Autodesk Inventor part; units mm, degrees
(part 4 of 6)
  line L2768 (19.2612, 25.2556) -> (20.2612, 25.2556)
  line L2769 (20.2612, 25.2556) -> (20.2612, 26.2556)
  line L2770 (20.2612, 26.2556) -> (19.2612, 26.2556)
  line L2771 (19.2612, 26.2556) -> (19.2612, 25.2556)
  line L2772 (19.8708, 25.2556) -> (20.8708, 25.2556)
  line L2773 (20.8708, 25.2556) -> (20.8708, 26.2556)
  line L2774 (20.8708, 26.2556) -> (19.8708, 26.2556)
  line L2775 (19.8708, 26.2556) -> (19.8708, 25.2556)
  line L2776 (20.4804, 25.2556) -> (21.4804, 25.2556)
  line L2777 (21.4804, 25.2556) -> (21.4804, 26.2556)
  line L2778 (21.4804, 26.2556) -> (20.4804, 26.2556)
  line L2779 (20.4804, 26.2556) -> (20.4804, 25.2556)
  line L2780 (21.2678, 25.2556) -> (22.2678, 25.2556)
  line L2781 (22.2678, 25.2556) -> (22.2678, 26.2556)
  line L2782 (22.2678, 26.2556) -> (21.2678, 26.2556)
  line L2783 (21.2678, 26.2556) -> (21.2678, 25.2556)
  line L2784 (21.7504, 25.2556) -> (22.7504, 25.2556)
  line L2785 (22.7504, 25.2556) -> (22.7504, 26.2556)
  line L2786 (22.7504, 26.2556) -> (21.7504, 26.2556)
  line L2787 (21.7504, 26.2556) -> (21.7504, 25.2556)
  line L2788 (12.8731, 25.281) -> (13.8731, 25.281)
  line L2789 (13.8731, 25.281) -> (13.8731, 26.281)
  line L2790 (13.8731, 26.281) -> (12.8731, 26.281)
  line L2791 (12.8731, 26.281) -> (12.8731, 25.281)
  line L2792 (14.5749, 25.281) -> (15.5749, 25.281)
  line L2793 (15.5749, 25.281) -> (15.5749, 26.281)
  line L2794 (15.5749, 26.281) -> (14.5749, 26.281)
  line L2795 (14.5749, 26.281) -> (14.5749, 25.281)
  line L2796 (15.4893, 25.281) -> (16.4893, 25.281)
  line L2797 (16.4893, 25.281) -> (16.4893, 26.281)
  line L2798 (16.4893, 26.281) -> (15.4893, 26.281)
  line L2799 (15.4893, 26.281) -> (15.4893, 25.281)
  line L2800 (16.2386, 25.281) -> (17.2386, 25.281)
  line L2801 (17.2386, 25.281) -> (17.2386, 26.281)
  line L2802 (17.2386, 26.281) -> (16.2386, 26.281)
  line L2803 (16.2386, 26.281) -> (16.2386, 25.281)
  line L2804 (17.0768, 25.281) -> (18.0768, 25.281)
  line L2805 (18.0768, 25.281) -> (18.0768, 26.281)
  line L2806 (18.0768, 26.281) -> (17.0768, 26.281)
  line L2807 (17.0768, 26.281) -> (17.0768, 25.281)
  line L2808 (17.9658, 25.281) -> (18.9658, 25.281)
  line L2809 (18.9658, 25.281) -> (18.9658, 26.281)
  line L2810 (18.9658, 26.281) -> (17.9658, 26.281)
  line L2811 (17.9658, 26.281) -> (17.9658, 25.281)
  line L2812 (18.6897, 25.281) -> (19.6897, 25.281)
  line L2813 (19.6897, 25.281) -> (19.6897, 26.281)
  line L2814 (19.6897, 26.281) -> (18.6897, 26.281)
  line L2815 (18.6897, 26.281) -> (18.6897, 25.281)
  line L2816 (19.2739, 25.281) -> (20.2739, 25.281)
  line L2817 (20.2739, 25.281) -> (20.2739, 26.281)
  line L2818 (20.2739, 26.281) -> (19.2739, 26.281)
  line L2819 (19.2739, 26.281) -> (19.2739, 25.281)
  line L2820 (19.8708, 25.281) -> (20.8708, 25.281)
  line L2821 (20.8708, 25.281) -> (20.8708, 26.281)
  line L2822 (20.8708, 26.281) -> (19.8708, 26.281)
  line L2823 (19.8708, 26.281) -> (19.8708, 25.281)
  line L2824 (20.4804, 25.281) -> (21.4804, 25.281)
  line L2825 (21.4804, 25.281) -> (21.4804, 26.281)
  line L2826 (21.4804, 26.281) -> (20.4804, 26.281)
  line L2827 (20.4804, 26.281) -> (20.4804, 25.281)
  line L2828 (21.2424, 25.281) -> (22.2424, 25.281)
  line L2829 (22.2424, 25.281) -> (22.2424, 26.281)
  line L2830 (22.2424, 26.281) -> (21.2424, 26.281)
  line L2831 (21.2424, 26.281) -> (21.2424, 25.281)
  line L2832 (21.7758, 25.281) -> (22.7758, 25.281)
  line L2833 (22.7758, 25.281) -> (22.7758, 26.281)
  line L2834 (22.7758, 26.281) -> (21.7758, 26.281)
  line L2835 (21.7758, 26.281) -> (21.7758, 25.281)
  line L2836 (12.8985, 25.3064) -> (13.8985, 25.3064)
  line L2837 (13.8985, 25.3064) -> (13.8985, 26.3064)
  line L2838 (13.8985, 26.3064) -> (12.8985, 26.3064)
  line L2839 (12.8985, 26.3064) -> (12.8985, 25.3064)
  line L2840 (14.6003, 25.3064) -> (15.6003, 25.3064)
  line L2841 (15.6003, 25.3064) -> (15.6003, 26.3064)
  line L2842 (15.6003, 26.3064) -> (14.6003, 26.3064)
  line L2843 (14.6003, 26.3064) -> (14.6003, 25.3064)
  line L2844 (15.502, 25.3064) -> (16.502, 25.3064)
  line L2845 (16.502, 25.3064) -> (16.502, 26.3064)
  line L2846 (16.502, 26.3064) -> (15.502, 26.3064)
  line L2847 (15.502, 26.3064) -> (15.502, 25.3064)
  line L2848 (16.2386, 25.3064) -> (17.2386, 25.3064)
  line L2849 (17.2386, 25.3064) -> (17.2386, 26.3064)
  line L2850 (17.2386, 26.3064) -> (16.2386, 26.3064)
  line L2851 (16.2386, 26.3064) -> (16.2386, 25.3064)
  line L2852 (17.0768, 25.3064) -> (18.0768, 25.3064)
  line L2853 (18.0768, 25.3064) -> (18.0768, 26.3064)
  line L2854 (18.0768, 26.3064) -> (17.0768, 26.3064)
  line L2855 (17.0768, 26.3064) -> (17.0768, 25.3064)
  line L2856 (17.9658, 25.3064) -> (18.9658, 25.3064)
  line L2857 (18.9658, 25.3064) -> (18.9658, 26.3064)
  line L2858 (18.9658, 26.3064) -> (17.9658, 26.3064)
  line L2859 (17.9658, 26.3064) -> (17.9658, 25.3064)
  line L2860 (18.677, 25.3064) -> (19.677, 25.3064)
  line L2861 (19.677, 25.3064) -> (19.677, 26.3064)
  line L2862 (19.677, 26.3064) -> (18.677, 26.3064)
  line L2863 (18.677, 26.3064) -> (18.677, 25.3064)
  line L2864 (19.2739, 25.3064) -> (20.2739, 25.3064)
  line L2865 (20.2739, 25.3064) -> (20.2739, 26.3064)
  line L2866 (20.2739, 26.3064) -> (19.2739, 26.3064)
  line L2867 (19.2739, 26.3064) -> (19.2739, 25.3064)
  line L2868 (19.7057, 25.3064) -> (20.7057, 25.3064)
  line L2869 (20.7057, 25.3064) -> (20.7057, 26.3064)
  line L2870 (20.7057, 26.3064) -> (19.7057, 26.3064)
  line L2871 (19.7057, 26.3064) -> (19.7057, 25.3064)
  line L2872 (20.0486, 25.3064) -> (21.0486, 25.3064)
  line L2873 (21.0486, 25.3064) -> (21.0486, 26.3064)
  line L2874 (21.0486, 26.3064) -> (20.0486, 26.3064)
  line L2875 (20.0486, 26.3064) -> (20.0486, 25.3064)
  line L2876 (20.4804, 25.3064) -> (21.4804, 25.3064)
  line L2877 (21.4804, 25.3064) -> (21.4804, 26.3064)
  line L2878 (21.4804, 26.3064) -> (20.4804, 26.3064)
  line L2879 (20.4804, 26.3064) -> (20.4804, 25.3064)
  line L2880 (21.2424, 25.3064) -> (22.2424, 25.3064)
  line L2881 (22.2424, 25.3064) -> (22.2424, 26.3064)
  line L2882 (22.2424, 26.3064) -> (21.2424, 26.3064)
  line L2883 (21.2424, 26.3064) -> (21.2424, 25.3064)
  line L2884 (21.7758, 25.3064) -> (22.7758, 25.3064)
  line L2885 (22.7758, 25.3064) -> (22.7758, 26.3064)
  line L2886 (22.7758, 26.3064) -> (21.7758, 26.3064)
  line L2887 (21.7758, 26.3064) -> (21.7758, 25.3064)
  line L2888 (12.9239, 25.3318) -> (13.9239, 25.3318)
  line L2889 (13.9239, 25.3318) -> (13.9239, 26.3318)
  line L2890 (13.9239, 26.3318) -> (12.9239, 26.3318)
  line L2891 (12.9239, 26.3318) -> (12.9239, 25.3318)
  line L2892 (14.6257, 25.3318) -> (15.6257, 25.3318)
  line L2893 (15.6257, 25.3318) -> (15.6257, 26.3318)
  line L2894 (15.6257, 26.3318) -> (14.6257, 26.3318)
  line L2895 (14.6257, 26.3318) -> (14.6257, 25.3318)
  line L2896 (15.502, 25.3318) -> (16.502, 25.3318)
  line L2897 (16.502, 25.3318) -> (16.502, 26.3318)
  line L2898 (16.502, 26.3318) -> (15.502, 26.3318)
  line L2899 (15.502, 26.3318) -> (15.502, 25.3318)
  line L2900 (16.2386, 25.3318) -> (17.2386, 25.3318)
  line L2901 (17.2386, 25.3318) -> (17.2386, 26.3318)
  line L2902 (17.2386, 26.3318) -> (16.2386, 26.3318)
  line L2903 (16.2386, 26.3318) -> (16.2386, 25.3318)
  line L2904 (17.0768, 25.3318) -> (18.0768, 25.3318)
  line L2905 (18.0768, 25.3318) -> (18.0768, 26.3318)
  line L2906 (18.0768, 26.3318) -> (17.0768, 26.3318)
  line L2907 (17.0768, 26.3318) -> (17.0768, 25.3318)
  line L2908 (17.9785, 25.3318) -> (18.9785, 25.3318)
  line L2909 (18.9785, 25.3318) -> (18.9785, 26.3318)
  line L2910 (18.9785, 26.3318) -> (17.9785, 26.3318)
  line L2911 (17.9785, 26.3318) -> (17.9785, 25.3318)
  line L2912 (18.6897, 25.3318) -> (19.6897, 25.3318)
  line L2913 (19.6897, 25.3318) -> (19.6897, 26.3318)
  line L2914 (19.6897, 26.3318) -> (18.6897, 26.3318)
  line L2915 (18.6897, 26.3318) -> (18.6897, 25.3318)
  line L2916 (19.2739, 25.3318) -> (20.2739, 25.3318)
  line L2917 (20.2739, 25.3318) -> (20.2739, 26.3318)
  line L2918 (20.2739, 26.3318) -> (19.2739, 26.3318)
  line L2919 (19.2739, 26.3318) -> (19.2739, 25.3318)
  line L2920 (19.693, 25.3318) -> (20.693, 25.3318)
  line L2921 (20.693, 25.3318) -> (20.693, 26.3318)
  line L2922 (20.693, 26.3318) -> (19.693, 26.3318)
  line L2923 (19.693, 26.3318) -> (19.693, 25.3318)
  line L2924 (20.0613, 25.3318) -> (21.0613, 25.3318)
  line L2925 (21.0613, 25.3318) -> (21.0613, 26.3318)
  line L2926 (21.0613, 26.3318) -> (20.0613, 26.3318)
  line L2927 (20.0613, 26.3318) -> (20.0613, 25.3318)
  line L2928 (20.4804, 25.3318) -> (21.4804, 25.3318)
  line L2929 (21.4804, 25.3318) -> (21.4804, 26.3318)
  line L2930 (21.4804, 26.3318) -> (20.4804, 26.3318)
  line L2931 (20.4804, 26.3318) -> (20.4804, 25.3318)
  line L2932 (21.2297, 25.3318) -> (22.2297, 25.3318)
  line L2933 (22.2297, 25.3318) -> (22.2297, 26.3318)
  line L2934 (22.2297, 26.3318) -> (21.2297, 26.3318)
  line L2935 (21.2297, 26.3318) -> (21.2297, 25.3318)
  line L2936 (21.8012, 25.3318) -> (22.8012, 25.3318)
  line L2937 (22.8012, 25.3318) -> (22.8012, 26.3318)
  line L2938 (22.8012, 26.3318) -> (21.8012, 26.3318)
  line L2939 (21.8012, 26.3318) -> (21.8012, 25.3318)
  line L2940 (12.9366, 25.3572) -> (13.9366, 25.3572)
  line L2941 (13.9366, 25.3572) -> (13.9366, 26.3572)
  line L2942 (13.9366, 26.3572) -> (12.9366, 26.3572)
  line L2943 (12.9366, 26.3572) -> (12.9366, 25.3572)
  line L2944 (14.6511, 25.3572) -> (15.6511, 25.3572)
  line L2945 (15.6511, 25.3572) -> (15.6511, 26.3572)
  line L2946 (15.6511, 26.3572) -> (14.6511, 26.3572)
  line L2947 (14.6511, 26.3572) -> (14.6511, 25.3572)
  line L2948 (15.502, 25.3572) -> (16.502, 25.3572)
  line L2949 (16.502, 25.3572) -> (16.502, 26.3572)
  line L2950 (16.502, 26.3572) -> (15.502, 26.3572)
  line L2951 (15.502, 26.3572) -> (15.502, 25.3572)
  line L2952 (16.2386, 25.3572) -> (17.2386, 25.3572)
  line L2953 (17.2386, 25.3572) -> (17.2386, 26.3572)
  line L2954 (17.2386, 26.3572) -> (16.2386, 26.3572)
  line L2955 (16.2386, 26.3572) -> (16.2386, 25.3572)
  line L2956 (16.7466, 25.3572) -> (17.7466, 25.3572)
  line L2957 (17.7466, 25.3572) -> (17.7466, 26.3572)
  line L2958 (17.7466, 26.3572) -> (16.7466, 26.3572)
  line L2959 (16.7466, 26.3572) -> (16.7466, 25.3572)
  line L2960 (17.4197, 25.3572) -> (18.4197, 25.3572)
  line L2961 (18.4197, 25.3572) -> (18.4197, 26.3572)
  line L2962 (18.4197, 26.3572) -> (17.4197, 26.3572)
  line L2963 (17.4197, 26.3572) -> (17.4197, 25.3572)
  line L2964 (17.9785, 25.3572) -> (18.9785, 25.3572)
  line L2965 (18.9785, 25.3572) -> (18.9785, 26.3572)
  line L2966 (18.9785, 26.3572) -> (17.9785, 26.3572)
  line L2967 (17.9785, 26.3572) -> (17.9785, 25.3572)
  line L2968 (18.6897, 25.3572) -> (19.6897, 25.3572)
  line L2969 (19.6897, 25.3572) -> (19.6897, 26.3572)
  line L2970 (19.6897, 26.3572) -> (18.6897, 26.3572)
  line L2971 (18.6897, 26.3572) -> (18.6897, 25.3572)
  line L2972 (19.2739, 25.3572) -> (20.2739, 25.3572)
  line L2973 (20.2739, 25.3572) -> (20.2739, 26.3572)
  line L2974 (20.2739, 26.3572) -> (19.2739, 26.3572)
  line L2975 (19.2739, 26.3572) -> (19.2739, 25.3572)
  line L2976 (19.693, 25.3572) -> (20.693, 25.3572)
  line L2977 (20.693, 25.3572) -> (20.693, 26.3572)
  line L2978 (20.693, 26.3572) -> (19.693, 26.3572)
  line L2979 (19.693, 26.3572) -> (19.693, 25.3572)
  line L2980 (20.0613, 25.3572) -> (21.0613, 25.3572)
  line L2981 (21.0613, 25.3572) -> (21.0613, 26.3572)
  line L2982 (21.0613, 26.3572) -> (20.0613, 26.3572)
  line L2983 (20.0613, 26.3572) -> (20.0613, 25.3572)
  line L2984 (20.4931, 25.3572) -> (21.4931, 25.3572)
  line L2985 (21.4931, 25.3572) -> (21.4931, 26.3572)
  line L2986 (21.4931, 26.3572) -> (20.4931, 26.3572)
  line L2987 (20.4931, 26.3572) -> (20.4931, 25.3572)
  line L2988 (21.217, 25.3572) -> (22.217, 25.3572)
  line L2989 (22.217, 25.3572) -> (22.217, 26.3572)
  line L2990 (22.217, 26.3572) -> (21.217, 26.3572)
  line L2991 (21.217, 26.3572) -> (21.217, 25.3572)
  line L2992 (21.8012, 25.3572) -> (22.8012, 25.3572)
  line L2993 (22.8012, 25.3572) -> (22.8012, 26.3572)
  line L2994 (22.8012, 26.3572) -> (21.8012, 26.3572)
  line L2995 (21.8012, 26.3572) -> (21.8012, 25.3572)
  line L2996 (12.962, 25.3826) -> (13.962, 25.3826)
  line L2997 (13.962, 25.3826) -> (13.962, 26.3826)
  line L2998 (13.962, 26.3826) -> (12.962, 26.3826)
  line L2999 (12.962, 26.3826) -> (12.962, 25.3826)
  line L3000 (14.6765, 25.3826) -> (15.6765, 25.3826)
  line L3001 (15.6765, 25.3826) -> (15.6765, 26.3826)
  line L3002 (15.6765, 26.3826) -> (14.6765, 26.3826)
  line L3003 (14.6765, 26.3826) -> (14.6765, 25.3826)
  line L3004 (15.5147, 25.3826) -> (16.5147, 25.3826)
  line L3005 (16.5147, 25.3826) -> (16.5147, 26.3826)
  line L3006 (16.5147, 26.3826) -> (15.5147, 26.3826)
  line L3007 (15.5147, 26.3826) -> (15.5147, 25.3826)
  line L3008 (16.2259, 25.3826) -> (17.2259, 25.3826)
  line L3009 (17.2259, 25.3826) -> (17.2259, 26.3826)
  line L3010 (17.2259, 26.3826) -> (16.2259, 26.3826)
  line L3011 (16.2259, 26.3826) -> (16.2259, 25.3826)
  line L3012 (16.7593, 25.3826) -> (17.7593, 25.3826)
  line L3013 (17.7593, 25.3826) -> (17.7593, 26.3826)
  line L3014 (17.7593, 26.3826) -> (16.7593, 26.3826)
  line L3015 (16.7593, 26.3826) -> (16.7593, 25.3826)
  line L3016 (17.4197, 25.3826) -> (18.4197, 25.3826)
  line L3017 (18.4197, 25.3826) -> (18.4197, 26.3826)
  line L3018 (18.4197, 26.3826) -> (17.4197, 26.3826)
  line L3019 (17.4197, 26.3826) -> (17.4197, 25.3826)
  line L3020 (17.9912, 25.3826) -> (18.9912, 25.3826)
  line L3021 (18.9912, 25.3826) -> (18.9912, 26.3826)
  line L3022 (18.9912, 26.3826) -> (17.9912, 26.3826)
  line L3023 (17.9912, 26.3826) -> (17.9912, 25.3826)
  line L3024 (18.6897, 25.3826) -> (19.6897, 25.3826)
  line L3025 (19.6897, 25.3826) -> (19.6897, 26.3826)
  line L3026 (19.6897, 26.3826) -> (18.6897, 26.3826)
  line L3027 (18.6897, 26.3826) -> (18.6897, 25.3826)
  line L3028 (19.2739, 25.3826) -> (20.2739, 25.3826)
  line L3029 (20.2739, 25.3826) -> (20.2739, 26.3826)
  line L3030 (20.2739, 26.3826) -> (19.2739, 26.3826)
  line L3031 (19.2739, 26.3826) -> (19.2739, 25.3826)
  line L3032 (19.693, 25.3826) -> (20.693, 25.3826)
  line L3033 (20.693, 25.3826) -> (20.693, 26.3826)
  line L3034 (20.693, 26.3826) -> (19.693, 26.3826)
  line L3035 (19.693, 26.3826) -> (19.693, 25.3826)
  line L3036 (20.0613, 25.3826) -> (21.0613, 25.3826)
  line L3037 (21.0613, 25.3826) -> (21.0613, 26.3826)
  line L3038 (21.0613, 26.3826) -> (20.0613, 26.3826)
  line L3039 (20.0613, 26.3826) -> (20.0613, 25.3826)
  line L3040 (20.4931, 25.3826) -> (21.4931, 25.3826)
  line L3041 (21.4931, 25.3826) -> (21.4931, 26.3826)
  line L3042 (21.4931, 26.3826) -> (20.4931, 26.3826)
  line L3043 (20.4931, 26.3826) -> (20.4931, 25.3826)
  line L3044 (21.217, 25.3826) -> (22.217, 25.3826)
  line L3045 (22.217, 25.3826) -> (22.217, 26.3826)
  line L3046 (22.217, 26.3826) -> (21.217, 26.3826)
  line L3047 (21.217, 26.3826) -> (21.217, 25.3826)
  line L3048 (21.8266, 25.3826) -> (22.8266, 25.3826)
  line L3049 (22.8266, 25.3826) -> (22.8266, 26.3826)
  line L3050 (22.8266, 26.3826) -> (21.8266, 26.3826)
  line L3051 (21.8266, 26.3826) -> (21.8266, 25.3826)
  line L3052 (12.9874, 25.408) -> (13.9874, 25.408)
  line L3053 (13.9874, 25.408) -> (13.9874, 26.408)
  line L3054 (13.9874, 26.408) -> (12.9874, 26.408)
  line L3055 (12.9874, 26.408) -> (12.9874, 25.408)
  line L3056 (14.7019, 25.408) -> (15.7019, 25.408)
  line L3057 (15.7019, 25.408) -> (15.7019, 26.408)
  line L3058 (15.7019, 26.408) -> (14.7019, 26.408)
  line L3059 (14.7019, 26.408) -> (14.7019, 25.408)
  line L3060 (15.5147, 25.408) -> (16.5147, 25.408)
  line L3061 (16.5147, 25.408) -> (16.5147, 26.408)
  line L3062 (16.5147, 26.408) -> (15.5147, 26.408)
  line L3063 (15.5147, 26.408) -> (15.5147, 25.408)
  line L3064 (16.2132, 25.408) -> (17.2132, 25.408)
  line L3065 (17.2132, 25.408) -> (17.2132, 26.408)
  line L3066 (17.2132, 26.408) -> (16.2132, 26.408)
  line L3067 (16.2132, 26.408) -> (16.2132, 25.408)
  line L3068 (16.7593, 25.408) -> (17.7593, 25.408)
  line L3069 (17.7593, 25.408) -> (17.7593, 26.408)
  line L3070 (17.7593, 26.408) -> (16.7593, 26.408)
  line L3071 (16.7593, 26.408) -> (16.7593, 25.408)
  line L3072 (17.4197, 25.408) -> (18.4197, 25.408)
  line L3073 (18.4197, 25.408) -> (18.4197, 26.408)
  line L3074 (18.4197, 26.408) -> (17.4197, 26.408)
  line L3075 (17.4197, 26.408) -> (17.4197, 25.408)
  line L3076 (18.0039, 25.408) -> (19.0039, 25.408)
  line L3077 (19.0039, 25.408) -> (19.0039, 26.408)
  line L3078 (19.0039, 26.408) -> (18.0039, 26.408)
  line L3079 (18.0039, 26.408) -> (18.0039, 25.408)
  line L3080 (18.677, 25.408) -> (19.677, 25.408)
  line L3081 (19.677, 25.408) -> (19.677, 26.408)
  line L3082 (19.677, 26.408) -> (18.677, 26.408)
  line L3083 (18.677, 26.408) -> (18.677, 25.408)
  line L3084 (19.2739, 25.408) -> (20.2739, 25.408)
  line L3085 (20.2739, 25.408) -> (20.2739, 26.408)
  line L3086 (20.2739, 26.408) -> (19.2739, 26.408)
  line L3087 (19.2739, 26.408) -> (19.2739, 25.408)
  line L3088 (19.693, 25.408) -> (20.693, 25.408)
  line L3089 (20.693, 25.408) -> (20.693, 26.408)
  line L3090 (20.693, 26.408) -> (19.693, 26.408)
  line L3091 (19.693, 26.408) -> (19.693, 25.408)
  line L3092 (20.0867, 25.408) -> (21.0867, 25.408)
  line L3093 (21.0867, 25.408) -> (21.0867, 26.408)
  line L3094 (21.0867, 26.408) -> (20.0867, 26.408)
  line L3095 (20.0867, 26.408) -> (20.0867, 25.408)
  line L3096 (20.4931, 25.408) -> (21.4931, 25.408)
  line L3097 (21.4931, 25.408) -> (21.4931, 26.408)
  line L3098 (21.4931, 26.408) -> (20.4931, 26.408)
  line L3099 (20.4931, 26.408) -> (20.4931, 25.408)
  line L3100 (21.2043, 25.408) -> (22.2043, 25.408)
  line L3101 (22.2043, 25.408) -> (22.2043, 26.408)
  line L3102 (22.2043, 26.408) -> (21.2043, 26.408)
  line L3103 (21.2043, 26.408) -> (21.2043, 25.408)
  line L3104 (21.8266, 25.408) -> (22.8266, 25.408)
  line L3105 (22.8266, 25.408) -> (22.8266, 26.408)
  line L3106 (22.8266, 26.408) -> (21.8266, 26.408)
  line L3107 (21.8266, 26.408) -> (21.8266, 25.408)
  line L3108 (13.0128, 25.4334) -> (14.0128, 25.4334)
  line L3109 (14.0128, 25.4334) -> (14.0128, 26.4334)
  line L3110 (14.0128, 26.4334) -> (13.0128, 26.4334)
  line L3111 (13.0128, 26.4334) -> (13.0128, 25.4334)
  line L3112 (14.7273, 25.4334) -> (15.7273, 25.4334)
  line L3113 (15.7273, 25.4334) -> (15.7273, 26.4334)
  line L3114 (15.7273, 26.4334) -> (14.7273, 26.4334)
  line L3115 (14.7273, 26.4334) -> (14.7273, 25.4334)
  line L3116 (15.5147, 25.4334) -> (16.5147, 25.4334)
  line L3117 (16.5147, 25.4334) -> (16.5147, 26.4334)
  line L3118 (16.5147, 26.4334) -> (15.5147, 26.4334)
  line L3119 (15.5147, 26.4334) -> (15.5147, 25.4334)
  line L3120 (16.2005, 25.4334) -> (17.2005, 25.4334)
  line L3121 (17.2005, 25.4334) -> (17.2005, 26.4334)
  line L3122 (17.2005, 26.4334) -> (16.2005, 26.4334)
  line L3123 (16.2005, 26.4334) -> (16.2005, 25.4334)
  line L3124 (16.7593, 25.4334) -> (17.7593, 25.4334)
  line L3125 (17.7593, 25.4334) -> (17.7593, 26.4334)
  line L3126 (17.7593, 26.4334) -> (16.7593, 26.4334)
  line L3127 (16.7593, 26.4334) -> (16.7593, 25.4334)
  line L3128 (17.4197, 25.4334) -> (18.4197, 25.4334)
  line L3129 (18.4197, 25.4334) -> (18.4197, 26.4334)
  line L3130 (18.4197, 26.4334) -> (17.4197, 26.4334)
  line L3131 (17.4197, 26.4334) -> (17.4197, 25.4334)
  line L3132 (18.0166, 25.4334) -> (19.0166, 25.4334)
  line L3133 (19.0166, 25.4334) -> (19.0166, 26.4334)
  line L3134 (19.0166, 26.4334) -> (18.0166, 26.4334)
  line L3135 (18.0166, 26.4334) -> (18.0166, 25.4334)
  line L3136 (18.6643, 25.4334) -> (19.6643, 25.4334)
  line L3137 (19.6643, 25.4334) -> (19.6643, 26.4334)
  line L3138 (19.6643, 26.4334) -> (18.6643, 26.4334)
  line L3139 (18.6643, 26.4334) -> (18.6643, 25.4334)
  line L3140 (19.2739, 25.4334) -> (20.2739, 25.4334)
  line L3141 (20.2739, 25.4334) -> (20.2739, 26.4334)
  line L3142 (20.2739, 26.4334) -> (19.2739, 26.4334)
  line L3143 (19.2739, 26.4334) -> (19.2739, 25.4334)
  line L3144 (19.6676, 25.4334) -> (20.6676, 25.4334)
  line L3145 (20.6676, 25.4334) -> (20.6676, 26.4334)
  line L3146 (20.6676, 26.4334) -> (19.6676, 26.4334)
  line L3147 (19.6676, 26.4334) -> (19.6676, 25.4334)
  line L3148 (20.0867, 25.4334) -> (21.0867, 25.4334)
  line L3149 (21.0867, 25.4334) -> (21.0867, 26.4334)
  line L3150 (21.0867, 26.4334) -> (20.0867, 26.4334)
  line L3151 (20.0867, 26.4334) -> (20.0867, 25.4334)
  line L3152 (20.4931, 25.4334) -> (21.4931, 25.4334)
  line L3153 (21.4931, 25.4334) -> (21.4931, 26.4334)
  line L3154 (21.4931, 26.4334) -> (20.4931, 26.4334)
  line L3155 (20.4931, 26.4334) -> (20.4931, 25.4334)
  line L3156 (21.1916, 25.4334) -> (22.1916, 25.4334)
  line L3157 (22.1916, 25.4334) -> (22.1916, 26.4334)
  line L3158 (22.1916, 26.4334) -> (21.1916, 26.4334)
  line L3159 (21.1916, 26.4334) -> (21.1916, 25.4334)
  line L3160 (21.8393, 25.4334) -> (22.8393, 25.4334)
  line L3161 (22.8393, 25.4334) -> (22.8393, 26.4334)
  line L3162 (22.8393, 26.4334) -> (21.8393, 26.4334)
  line L3163 (21.8393, 26.4334) -> (21.8393, 25.4334)
  line L3164 (13.0255, 25.4588) -> (14.0255, 25.4588)
  line L3165 (14.0255, 25.4588) -> (14.0255, 26.4588)
  line L3166 (14.0255, 26.4588) -> (13.0255, 26.4588)
  line L3167 (13.0255, 26.4588) -> (13.0255, 25.4588)
  line L3168 (14.74, 25.4588) -> (15.74, 25.4588)
  line L3169 (15.74, 25.4588) -> (15.74, 26.4588)
  line L3170 (15.74, 26.4588) -> (14.74, 26.4588)
  line L3171 (14.74, 26.4588) -> (14.74, 25.4588)
  line L3172 (15.5147, 25.4588) -> (16.5147, 25.4588)
  line L3173 (16.5147, 25.4588) -> (16.5147, 26.4588)
  line L3174 (16.5147, 26.4588) -> (15.5147, 26.4588)
  line L3175 (15.5147, 26.4588) -> (15.5147, 25.4588)
  line L3176 (16.1878, 25.4588) -> (17.1878, 25.4588)
  line L3177 (17.1878, 25.4588) -> (17.1878, 26.4588)
  line L3178 (17.1878, 26.4588) -> (16.1878, 26.4588)
  line L3179 (16.1878, 26.4588) -> (16.1878, 25.4588)
  line L3180 (16.7847, 25.4588) -> (17.7847, 25.4588)
  line L3181 (17.7847, 25.4588) -> (17.7847, 26.4588)
  line L3182 (17.7847, 26.4588) -> (16.7847, 26.4588)
  line L3183 (16.7847, 26.4588) -> (16.7847, 25.4588)
  line L3184 (17.4197, 25.4588) -> (18.4197, 25.4588)
  line L3185 (18.4197, 25.4588) -> (18.4197, 26.4588)
  line L3186 (18.4197, 26.4588) -> (17.4197, 26.4588)
  line L3187 (17.4197, 26.4588) -> (17.4197, 25.4588)
  line L3188 (18.3341, 25.4588) -> (19.3341, 25.4588)
  line L3189 (19.3341, 25.4588) -> (19.3341, 26.4588)
  line L3190 (19.3341, 26.4588) -> (18.3341, 26.4588)
  line L3191 (18.3341, 26.4588) -> (18.3341, 25.4588)
  line L3192 (19.2739, 25.4588) -> (20.2739, 25.4588)
  line L3193 (20.2739, 25.4588) -> (20.2739, 26.4588)
  line L3194 (20.2739, 26.4588) -> (19.2739, 26.4588)
  line L3195 (19.2739, 26.4588) -> (19.2739, 25.4588)
  line L3196 (19.6676, 25.4588) -> (20.6676, 25.4588)
  line L3197 (20.6676, 25.4588) -> (20.6676, 26.4588)
  line L3198 (20.6676, 26.4588) -> (19.6676, 26.4588)
  line L3199 (19.6676, 26.4588) -> (19.6676, 25.4588)
  line L3200 (20.0867, 25.4588) -> (21.0867, 25.4588)
  line L3201 (21.0867, 25.4588) -> (21.0867, 26.4588)
  line L3202 (21.0867, 26.4588) -> (20.0867, 26.4588)
  line L3203 (20.0867, 26.4588) -> (20.0867, 25.4588)
  line L3204 (20.4931, 25.4588) -> (21.4931, 25.4588)
  line L3205 (21.4931, 25.4588) -> (21.4931, 26.4588)
  line L3206 (21.4931, 26.4588) -> (20.4931, 26.4588)
  line L3207 (20.4931, 26.4588) -> (20.4931, 25.4588)
  line L3208 (21.1916, 25.4588) -> (22.1916, 25.4588)
  line L3209 (22.1916, 25.4588) -> (22.1916, 26.4588)
  line L3210 (22.1916, 26.4588) -> (21.1916, 26.4588)
  line L3211 (21.1916, 26.4588) -> (21.1916, 25.4588)
  line L3212 (21.852, 25.4588) -> (22.852, 25.4588)
  line L3213 (22.852, 25.4588) -> (22.852, 26.4588)
  line L3214 (22.852, 26.4588) -> (21.852, 26.4588)
  line L3215 (21.852, 26.4588) -> (21.852, 25.4588)
  line L3216 (12.4667, 25.4842) -> (13.4667, 25.4842)
  line L3217 (13.4667, 25.4842) -> (13.4667, 26.4842)
  line L3218 (13.4667, 26.4842) -> (12.4667, 26.4842)
  line L3219 (12.4667, 26.4842) -> (12.4667, 25.4842)
  line L3220 (13.0509, 25.4842) -> (14.0509, 25.4842)
  line L3221 (14.0509, 25.4842) -> (14.0509, 26.4842)
  line L3222 (14.0509, 26.4842) -> (13.0509, 26.4842)
  line L3223 (13.0509, 26.4842) -> (13.0509, 25.4842)
  line L3224 (14.7654, 25.4842) -> (15.7654, 25.4842)
  line L3225 (15.7654, 25.4842) -> (15.7654, 26.4842)
  line L3226 (15.7654, 26.4842) -> (14.7654, 26.4842)
  line L3227 (14.7654, 26.4842) -> (14.7654, 25.4842)
  line L3228 (15.5528, 25.4842) -> (16.5528, 25.4842)
  line L3229 (16.5528, 25.4842) -> (16.5528, 26.4842)
  line L3230 (16.5528, 26.4842) -> (15.5528, 26.4842)
  line L3231 (15.5528, 26.4842) -> (15.5528, 25.4842)
  line L3232 (16.1497, 25.4842) -> (17.1497, 25.4842)
  line L3233 (17.1497, 25.4842) -> (17.1497, 26.4842)
  line L3234 (17.1497, 26.4842) -> (16.1497, 26.4842)
  line L3235 (16.1497, 26.4842) -> (16.1497, 25.4842)
  line L3236 (16.7974, 25.4842) -> (17.7974, 25.4842)
  line L3237 (17.7974, 25.4842) -> (17.7974, 26.4842)
  line L3238 (17.7974, 26.4842) -> (16.7974, 26.4842)
  line L3239 (16.7974, 26.4842) -> (16.7974, 25.4842)
  line L3240 (17.3943, 25.4842) -> (18.3943, 25.4842)
  line L3241 (18.3943, 25.4842) -> (18.3943, 26.4842)
  line L3242 (18.3943, 26.4842) -> (17.3943, 26.4842)
  line L3243 (17.3943, 26.4842) -> (17.3943, 25.4842)
  line L3244 (18.3341, 25.4842) -> (19.3341, 25.4842)
  line L3245 (19.3341, 25.4842) -> (19.3341, 26.4842)
  line L3246 (19.3341, 26.4842) -> (18.3341, 26.4842)
  line L3247 (18.3341, 26.4842) -> (18.3341, 25.4842)
  line L3248 (19.2739, 25.4842) -> (20.2739, 25.4842)
  line L3249 (20.2739, 25.4842) -> (20.2739, 26.4842)
  line L3250 (20.2739, 26.4842) -> (19.2739, 26.4842)
  line L3251 (19.2739, 26.4842) -> (19.2739, 25.4842)
  line L3252 (19.6676, 25.4842) -> (20.6676, 25.4842)
  line L3253 (20.6676, 25.4842) -> (20.6676, 26.4842)
  line L3254 (20.6676, 26.4842) -> (19.6676, 26.4842)
  line L3255 (19.6676, 26.4842) -> (19.6676, 25.4842)
  line L3256 (20.1121, 25.4842) -> (21.1121, 25.4842)
  line L3257 (21.1121, 25.4842) -> (21.1121, 26.4842)
  line L3258 (21.1121, 26.4842) -> (20.1121, 26.4842)
  line L3259 (20.1121, 26.4842) -> (20.1121, 25.4842)
  line L3260 (20.4931, 25.4842) -> (21.4931, 25.4842)
  line L3261 (21.4931, 25.4842) -> (21.4931, 26.4842)
  line L3262 (21.4931, 26.4842) -> (20.4931, 26.4842)
  line L3263 (20.4931, 26.4842) -> (20.4931, 25.4842)
  line L3264 (21.1789, 25.4842) -> (22.1789, 25.4842)
  line L3265 (22.1789, 25.4842) -> (22.1789, 26.4842)
  line L3266 (22.1789, 26.4842) -> (21.1789, 26.4842)
  line L3267 (21.1789, 26.4842) -> (21.1789, 25.4842)
  line L3268 (21.8647, 25.4842) -> (22.8647, 25.4842)
  line L3269 (22.8647, 25.4842) -> (22.8647, 26.4842)
  line L3270 (22.8647, 26.4842) -> (21.8647, 26.4842)
  line L3271 (21.8647, 26.4842) -> (21.8647, 25.4842)
  line L3272 (12.4921, 25.5096) -> (13.4921, 25.5096)
  line L3273 (13.4921, 25.5096) -> (13.4921, 26.5096)
  line L3274 (13.4921, 26.5096) -> (12.4921, 26.5096)
  line L3275 (12.4921, 26.5096) -> (12.4921, 25.5096)
  line L3276 (13.0763, 25.5096) -> (14.0763, 25.5096)
  line L3277 (14.0763, 25.5096) -> (14.0763, 26.5096)
  line L3278 (14.0763, 26.5096) -> (13.0763, 26.5096)
  line L3279 (13.0763, 26.5096) -> (13.0763, 25.5096)
  line L3280 (14.7908, 25.5096) -> (15.7908, 25.5096)
  line L3281 (15.7908, 25.5096) -> (15.7908, 26.5096)
  line L3282 (15.7908, 26.5096) -> (14.7908, 26.5096)
  line L3283 (14.7908, 26.5096) -> (14.7908, 25.5096)
  line L3284 (15.8576, 25.5096) -> (16.8576, 25.5096)
  line L3285 (16.8576, 25.5096) -> (16.8576, 26.5096)
  line L3286 (16.8576, 26.5096) -> (15.8576, 26.5096)
  line L3287 (15.8576, 26.5096) -> (15.8576, 25.5096)
  line L3288 (16.8228, 25.5096) -> (17.8228, 25.5096)
  line L3289 (17.8228, 25.5096) -> (17.8228, 26.5096)
  line L3290 (17.8228, 26.5096) -> (16.8228, 26.5096)
  line L3291 (16.8228, 26.5096) -> (16.8228, 25.5096)
  line L3292 (17.3943, 25.5096) -> (18.3943, 25.5096)
  line L3293 (18.3943, 25.5096) -> (18.3943, 26.5096)
  line L3294 (18.3943, 26.5096) -> (17.3943, 26.5096)
  line L3295 (17.3943, 26.5096) -> (17.3943, 25.5096)
  line L3296 (18.3341, 25.5096) -> (19.3341, 25.5096)
  line L3297 (19.3341, 25.5096) -> (19.3341, 26.5096)
  line L3298 (19.3341, 26.5096) -> (18.3341, 26.5096)
  line L3299 (18.3341, 26.5096) -> (18.3341, 25.5096)
  line L3300 (19.2739, 25.5096) -> (20.2739, 25.5096)
  line L3301 (20.2739, 25.5096) -> (20.2739, 26.5096)
  line L3302 (20.2739, 26.5096) -> (19.2739, 26.5096)
  line L3303 (19.2739, 26.5096) -> (19.2739, 25.5096)
  line L3304 (19.6676, 25.5096) -> (20.6676, 25.5096)
  line L3305 (20.6676, 25.5096) -> (20.6676, 26.5096)
  line L3306 (20.6676, 26.5096) -> (19.6676, 26.5096)
  line L3307 (19.6676, 26.5096) -> (19.6676, 25.5096)
  line L3308 (20.1121, 25.5096) -> (21.1121, 25.5096)
  line L3309 (21.1121, 25.5096) -> (21.1121, 26.5096)
  line L3310 (21.1121, 26.5096) -> (20.1121, 26.5096)
  line L3311 (20.1121, 26.5096) -> (20.1121, 25.5096)
  line L3312 (20.4931, 25.5096) -> (21.4931, 25.5096)
  line L3313 (21.4931, 25.5096) -> (21.4931, 26.5096)
  line L3314 (21.4931, 26.5096) -> (20.4931, 26.5096)
  line L3315 (20.4931, 26.5096) -> (20.4931, 25.5096)
  line L3316 (21.1789, 25.5096) -> (22.1789, 25.5096)
  line L3317 (22.1789, 25.5096) -> (22.1789, 26.5096)
  line L3318 (22.1789, 26.5096) -> (21.1789, 26.5096)
  line L3319 (21.1789, 26.5096) -> (21.1789, 25.5096)
  line L3320 (21.8774, 25.5096) -> (22.8774, 25.5096)
  line L3321 (22.8774, 25.5096) -> (22.8774, 26.5096)
  line L3322 (22.8774, 26.5096) -> (21.8774, 26.5096)
  line L3323 (21.8774, 26.5096) -> (21.8774, 25.5096)
  line L3324 (12.5175, 25.535) -> (13.5175, 25.535)
  line L3325 (13.5175, 25.535) -> (13.5175, 26.535)
  line L3326 (13.5175, 26.535) -> (12.5175, 26.535)
  line L3327 (12.5175, 26.535) -> (12.5175, 25.535)
  line L3328 (13.1017, 25.535) -> (14.1017, 25.535)
  line L3329 (14.1017, 25.535) -> (14.1017, 26.535)
  line L3330 (14.1017, 26.535) -> (13.1017, 26.535)
  line L3331 (13.1017, 26.535) -> (13.1017, 25.535)
  line L3332 (14.8162, 25.535) -> (15.8162, 25.535)
  line L3333 (15.8162, 25.535) -> (15.8162, 26.535)
  line L3334 (15.8162, 26.535) -> (14.8162, 26.535)
  line L3335 (14.8162, 26.535) -> (14.8162, 25.535)
  line L3336 (15.8449, 25.535) -> (16.8449, 25.535)
  line L3337 (16.8449, 25.535) -> (16.8449, 26.535)
  line L3338 (16.8449, 26.535) -> (15.8449, 26.535)
  line L3339 (15.8449, 26.535) -> (15.8449, 25.535)
  line L3340 (16.8482, 25.535) -> (17.8482, 25.535)
  line L3341 (17.8482, 25.535) -> (17.8482, 26.535)
  line L3342 (17.8482, 26.535) -> (16.8482, 26.535)
  line L3343 (16.8482, 26.535) -> (16.8482, 25.535)
  line L3344 (17.3689, 25.535) -> (18.3689, 25.535)
  line L3345 (18.3689, 25.535) -> (18.3689, 26.535)
  line L3346 (18.3689, 26.535) -> (17.3689, 26.535)
  line L3347 (17.3689, 26.535) -> (17.3689, 25.535)
  line L3348 (18.3214, 25.535) -> (19.3214, 25.535)
  line L3349 (19.3214, 25.535) -> (19.3214, 26.535)
  line L3350 (19.3214, 26.535) -> (18.3214, 26.535)
  line L3351 (18.3214, 26.535) -> (18.3214, 25.535)
  line L3352 (19.2739, 25.535) -> (20.2739, 25.535)
  line L3353 (20.2739, 25.535) -> (20.2739, 26.535)
  line L3354 (20.2739, 26.535) -> (19.2739, 26.535)
  line L3355 (19.2739, 26.535) -> (19.2739, 25.535)
  line L3356 (19.6549, 25.535) -> (20.6549, 25.535)
  line L3357 (20.6549, 25.535) -> (20.6549, 26.535)
  line L3358 (20.6549, 26.535) -> (19.6549, 26.535)
  line L3359 (19.6549, 26.535) -> (19.6549, 25.535)
  line L3360 (20.1121, 25.535) -> (21.1121, 25.535)
  line L3361 (21.1121, 25.535) -> (21.1121, 26.535)
  line L3362 (21.1121, 26.535) -> (20.1121, 26.535)
  line L3363 (20.1121, 26.535) -> (20.1121, 25.535)
  line L3364 (20.4931, 25.535) -> (21.4931, 25.535)
  line L3365 (21.4931, 25.535) -> (21.4931, 26.535)
  line L3366 (21.4931, 26.535) -> (20.4931, 26.535)
  line L3367 (20.4931, 26.535) -> (20.4931, 25.535)
  line L3368 (21.1662, 25.535) -> (22.1662, 25.535)
  line L3369 (22.1662, 25.535) -> (22.1662, 26.535)
  line L3370 (22.1662, 26.535) -> (21.1662, 26.535)
  line L3371 (21.1662, 26.535) -> (21.1662, 25.535)
  line L3372 (21.8901, 25.535) -> (22.8901, 25.535)
  line L3373 (22.8901, 25.535) -> (22.8901, 26.535)
  line L3374 (22.8901, 26.535) -> (21.8901, 26.535)
  line L3375 (21.8901, 26.535) -> (21.8901, 25.535)
  line L3376 (12.5302, 25.5604) -> (13.5302, 25.5604)
  line L3377 (13.5302, 25.5604) -> (13.5302, 26.5604)
  line L3378 (13.5302, 26.5604) -> (12.5302, 26.5604)
  line L3379 (12.5302, 26.5604) -> (12.5302, 25.5604)
  line L3380 (13.1144, 25.5604) -> (14.1144, 25.5604)
  line L3381 (14.1144, 25.5604) -> (14.1144, 26.5604)
  line L3382 (14.1144, 26.5604) -> (13.1144, 26.5604)
  line L3383 (13.1144, 26.5604) -> (13.1144, 25.5604)
  line L3384 (14.7447, 26.0477) -> (14.7701, 26.0477)
  line L3385 (14.7701, 26.0477) -> (14.7701, 26.0731)
  line L3386 (14.7701, 26.0731) -> (14.7447, 26.0731)
  line L3387 (14.7447, 26.0731) -> (14.7447, 26.0477)
  line L3388 (14.8289, 25.5604) -> (15.8289, 25.5604)
  line L3389 (15.8289, 25.5604) -> (15.8289, 26.5604)
  line L3390 (15.8289, 26.5604) -> (14.8289, 26.5604)
  line L3391 (14.8289, 26.5604) -> (14.8289, 25.5604)
  line L3392 (15.8449, 25.5604) -> (16.8449, 25.5604)
  line L3393 (16.8449, 25.5604) -> (16.8449, 26.5604)
  line L3394 (16.8449, 26.5604) -> (15.8449, 26.5604)
  line L3395 (15.8449, 26.5604) -> (15.8449, 25.5604)
  line L3396 (17.1022, 25.5604) -> (18.1022, 25.5604)
  line L3397 (18.1022, 25.5604) -> (18.1022, 26.5604)
  line L3398 (18.1022, 26.5604) -> (17.1022, 26.5604)
  line L3399 (17.1022, 26.5604) -> (17.1022, 25.5604)
  line L3400 (18.3214, 25.5604) -> (19.3214, 25.5604)
  line L3401 (19.3214, 25.5604) -> (19.3214, 26.5604)
  line L3402 (19.3214, 26.5604) -> (18.3214, 26.5604)
  line L3403 (18.3214, 26.5604) -> (18.3214, 25.5604)
  line L3404 (19.2993, 25.5604) -> (20.2993, 25.5604)
  line L3405 (20.2993, 25.5604) -> (20.2993, 26.5604)
  line L3406 (20.2993, 26.5604) -> (19.2993, 26.5604)
  line L3407 (19.2993, 26.5604) -> (19.2993, 25.5604)
  line L3408 (19.6422, 25.5604) -> (20.6422, 25.5604)
  line L3409 (20.6422, 25.5604) -> (20.6422, 26.5604)
  line L3410 (20.6422, 26.5604) -> (19.6422, 26.5604)
  line L3411 (19.6422, 26.5604) -> (19.6422, 25.5604)
  line L3412 (20.1375, 25.5604) -> (21.1375, 25.5604)
  line L3413 (21.1375, 25.5604) -> (21.1375, 26.5604)
  line L3414 (21.1375, 26.5604) -> (20.1375, 26.5604)
  line L3415 (20.1375, 26.5604) -> (20.1375, 25.5604)
  line L3416 (20.5058, 25.5604) -> (21.5058, 25.5604)
  line L3417 (21.5058, 25.5604) -> (21.5058, 26.5604)
  line L3418 (21.5058, 26.5604) -> (20.5058, 26.5604)
  line L3419 (20.5058, 26.5604) -> (20.5058, 25.5604)
  line L3420 (21.1535, 25.5604) -> (22.1535, 25.5604)
  line L3421 (22.1535, 25.5604) -> (22.1535, 26.5604)
  line L3422 (22.1535, 26.5604) -> (21.1535, 26.5604)
  line L3423 (21.1535, 26.5604) -> (21.1535, 25.5604)
  line L3424 (21.9028, 25.5604) -> (22.9028, 25.5604)
  line L3425 (22.9028, 25.5604) -> (22.9028, 26.5604)
  line L3426 (22.9028, 26.5604) -> (21.9028, 26.5604)
  line L3427 (21.9028, 26.5604) -> (21.9028, 25.5604)
  line L3428 (12.5556, 25.5858) -> (13.5556, 25.5858)
  line L3429 (13.5556, 25.5858) -> (13.5556, 26.5858)
  line L3430 (13.5556, 26.5858) -> (12.5556, 26.5858)
  line L3431 (12.5556, 26.5858) -> (12.5556, 25.5858)
  line L3432 (13.1398, 25.5858) -> (14.1398, 25.5858)
  line L3433 (14.1398, 25.5858) -> (14.1398, 26.5858)
  line L3434 (14.1398, 26.5858) -> (13.1398, 26.5858)
  line L3435 (13.1398, 26.5858) -> (13.1398, 25.5858)
  line L3436 (14.2701, 25.5858) -> (15.2701, 25.5858)
  line L3437 (15.2701, 25.5858) -> (15.2701, 26.5858)
  line L3438 (15.2701, 26.5858) -> (14.2701, 26.5858)
  line L3439 (14.2701, 26.5858) -> (14.2701, 25.5858)
  line L3440 (14.867, 25.5858) -> (15.867, 25.5858)
  line L3441 (15.867, 25.5858) -> (15.867, 26.5858)
  line L3442 (15.867, 26.5858) -> (14.867, 26.5858)
  line L3443 (14.867, 26.5858) -> (14.867, 25.5858)
  line L3444 (15.8322, 25.5858) -> (16.8322, 25.5858)
  line L3445 (16.8322, 25.5858) -> (16.8322, 26.5858)
  line L3446 (16.8322, 26.5858) -> (15.8322, 26.5858)
  line L3447 (15.8322, 26.5858) -> (15.8322, 25.5858)
  line L3448 (17.1149, 25.5858) -> (18.1149, 25.5858)
  line L3449 (18.1149, 25.5858) -> (18.1149, 26.5858)
  line L3450 (18.1149, 26.5858) -> (17.1149, 26.5858)
  line L3451 (17.1149, 26.5858) -> (17.1149, 25.5858)
  line L3452 (18.3214, 25.5858) -> (19.3214, 25.5858)
  line L3453 (19.3214, 25.5858) -> (19.3214, 26.5858)
  line L3454 (19.3214, 26.5858) -> (18.3214, 26.5858)
  line L3455 (18.3214, 26.5858) -> (18.3214, 25.5858)
  line L3456 (19.2993, 25.5858) -> (20.2993, 25.5858)
  line L3457 (20.2993, 25.5858) -> (20.2993, 26.5858)
  line L3458 (20.2993, 26.5858) -> (19.2993, 26.5858)
  line L3459 (19.2993, 26.5858) -> (19.2993, 25.5858)
  line L3460 (19.6422, 25.5858) -> (20.6422, 25.5858)
  line L3461 (20.6422, 25.5858) -> (20.6422, 26.5858)
  line L3462 (20.6422, 26.5858) -> (19.6422, 26.5858)
  line L3463 (19.6422, 26.5858) -> (19.6422, 25.5858)
  line L3464 (20.1375, 25.5858) -> (21.1375, 25.5858)
  line L3465 (21.1375, 25.5858) -> (21.1375, 26.5858)
  line L3466 (21.1375, 26.5858) -> (20.1375, 26.5858)
  line L3467 (20.1375, 26.5858) -> (20.1375, 25.5858)
  line L3468 (20.5058, 25.5858) -> (21.5058, 25.5858)
  line L3469 (21.5058, 25.5858) -> (21.5058, 26.5858)
  line L3470 (21.5058, 26.5858) -> (20.5058, 26.5858)
  line L3471 (20.5058, 26.5858) -> (20.5058, 25.5858)
  line L3472 (21.1535, 25.5858) -> (22.1535, 25.5858)
  line L3473 (22.1535, 25.5858) -> (22.1535, 26.5858)
  line L3474 (22.1535, 26.5858) -> (21.1535, 26.5858)
  line L3475 (21.1535, 26.5858) -> (21.1535, 25.5858)
  line L3476 (21.9155, 25.5858) -> (22.9155, 25.5858)
  line L3477 (22.9155, 25.5858) -> (22.9155, 26.5858)
  line L3478 (22.9155, 26.5858) -> (21.9155, 26.5858)
  line L3479 (21.9155, 26.5858) -> (21.9155, 25.5858)
  line L3480 (12.581, 25.6112) -> (13.581, 25.6112)
  line L3481 (13.581, 25.6112) -> (13.581, 26.6112)
  line L3482 (13.581, 26.6112) -> (12.581, 26.6112)
  line L3483 (12.581, 26.6112) -> (12.581, 25.6112)
  line L3484 (13.1652, 25.6112) -> (14.1652, 25.6112)
  line L3485 (14.1652, 25.6112) -> (14.1652, 26.6112)
  line L3486 (14.1652, 26.6112) -> (13.1652, 26.6112)
  line L3487 (13.1652, 26.6112) -> (13.1652, 25.6112)
  line L3488 (14.2955, 25.6112) -> (15.2955, 25.6112)
  line L3489 (15.2955, 25.6112) -> (15.2955, 26.6112)
  line L3490 (15.2955, 26.6112) -> (14.2955, 26.6112)
  line L3491 (14.2955, 26.6112) -> (14.2955, 25.6112)
  line L3492 (14.8924, 25.6112) -> (15.8924, 25.6112)
  line L3493 (15.8924, 25.6112) -> (15.8924, 26.6112)
  line L3494 (15.8924, 26.6112) -> (14.8924, 26.6112)
  line L3495 (14.8924, 26.6112) -> (14.8924, 25.6112)
  line L3496 (15.8195, 25.6112) -> (16.8195, 25.6112)
  line L3497 (16.8195, 25.6112) -> (16.8195, 26.6112)
  line L3498 (16.8195, 26.6112) -> (15.8195, 26.6112)
  line L3499 (15.8195, 26.6112) -> (15.8195, 25.6112)
  line L3500 (17.1022, 25.6112) -> (18.1022, 25.6112)
  line L3501 (18.1022, 25.6112) -> (18.1022, 26.6112)
  line L3502 (18.1022, 26.6112) -> (17.1022, 26.6112)
  line L3503 (17.1022, 26.6112) -> (17.1022, 25.6112)
  line L3504 (18.3087, 25.6112) -> (19.3087, 25.6112)
  line L3505 (19.3087, 25.6112) -> (19.3087, 26.6112)
  line L3506 (19.3087, 26.6112) -> (18.3087, 26.6112)
  line L3507 (18.3087, 26.6112) -> (18.3087, 25.6112)
  line L3508 (19.2993, 25.6112) -> (20.2993, 25.6112)
  line L3509 (20.2993, 25.6112) -> (20.2993, 26.6112)
  line L3510 (20.2993, 26.6112) -> (19.2993, 26.6112)
  line L3511 (19.2993, 26.6112) -> (19.2993, 25.6112)
  line L3512 (19.6422, 25.6112) -> (20.6422, 25.6112)
  line L3513 (20.6422, 25.6112) -> (20.6422, 26.6112)
  line L3514 (20.6422, 26.6112) -> (19.6422, 26.6112)
  line L3515 (19.6422, 26.6112) -> (19.6422, 25.6112)
  line L3516 (20.1375, 25.6112) -> (21.1375, 25.6112)
  line L3517 (21.1375, 25.6112) -> (21.1375, 26.6112)
  line L3518 (21.1375, 26.6112) -> (20.1375, 26.6112)
  line L3519 (20.1375, 26.6112) -> (20.1375, 25.6112)
  line L3520 (20.5058, 25.6112) -> (21.5058, 25.6112)
  line L3521 (21.5058, 25.6112) -> (21.5058, 26.6112)
  line L3522 (21.5058, 26.6112) -> (20.5058, 26.6112)
  line L3523 (20.5058, 26.6112) -> (20.5058, 25.6112)
  line L3524 (21.1408, 25.6112) -> (22.1408, 25.6112)
  line L3525 (22.1408, 25.6112) -> (22.1408, 26.6112)
  line L3526 (22.1408, 26.6112) -> (21.1408, 26.6112)
  line L3527 (21.1408, 26.6112) -> (21.1408, 25.6112)
  line L3528 (21.9282, 25.6112) -> (22.9282, 25.6112)
  line L3529 (22.9282, 25.6112) -> (22.9282, 26.6112)
  line L3530 (22.9282, 26.6112) -> (21.9282, 26.6112)
  line L3531 (21.9282, 26.6112) -> (21.9282, 25.6112)
  line L3532 (12.5937, 25.6366) -> (13.5937, 25.6366)
  line L3533 (13.5937, 25.6366) -> (13.5937, 26.6366)
  line L3534 (13.5937, 26.6366) -> (12.5937, 26.6366)
  line L3535 (12.5937, 26.6366) -> (12.5937, 25.6366)
  line L3536 (13.1779, 25.6366) -> (14.1779, 25.6366)
  line L3537 (14.1779, 25.6366) -> (14.1779, 26.6366)
  line L3538 (14.1779, 26.6366) -> (13.1779, 26.6366)
  line L3539 (13.1779, 26.6366) -> (13.1779, 25.6366)
  line L3540 (14.3209, 25.6366) -> (15.3209, 25.6366)
  line L3541 (15.3209, 25.6366) -> (15.3209, 26.6366)
  line L3542 (15.3209, 26.6366) -> (14.3209, 26.6366)
  line L3543 (14.3209, 26.6366) -> (14.3209, 25.6366)
  line L3544 (14.9178, 25.6366) -> (15.9178, 25.6366)
  line L3545 (15.9178, 25.6366) -> (15.9178, 26.6366)
  line L3546 (15.9178, 26.6366) -> (14.9178, 26.6366)
  line L3547 (14.9178, 26.6366) -> (14.9178, 25.6366)
  line L3548 (15.8068, 25.6366) -> (16.8068, 25.6366)
  line L3549 (16.8068, 25.6366) -> (16.8068, 26.6366)
  line L3550 (16.8068, 26.6366) -> (15.8068, 26.6366)
  line L3551 (15.8068, 26.6366) -> (15.8068, 25.6366)
  line L3552 (17.1022, 25.6366) -> (18.1022, 25.6366)
  line L3553 (18.1022, 25.6366) -> (18.1022, 26.6366)
  line L3554 (18.1022, 26.6366) -> (17.1022, 26.6366)
  line L3555 (17.1022, 26.6366) -> (17.1022, 25.6366)
  line L3556 (17.9658, 25.6366) -> (18.9658, 25.6366)
  line L3557 (18.9658, 25.6366) -> (18.9658, 26.6366)
  line L3558 (18.9658, 26.6366) -> (17.9658, 26.6366)
  line L3559 (17.9658, 26.6366) -> (17.9658, 25.6366)
  line L3560 (18.5119, 25.6366) -> (19.5119, 25.6366)
  line L3561 (19.5119, 25.6366) -> (19.5119, 26.6366)
  line L3562 (19.5119, 26.6366) -> (18.5119, 26.6366)
  line L3563 (18.5119, 26.6366) -> (18.5119, 25.6366)
  line L3564 (19.2993, 25.6366) -> (20.2993, 25.6366)
  line L3565 (20.2993, 25.6366) -> (20.2993, 26.6366)
  line L3566 (20.2993, 26.6366) -> (19.2993, 26.6366)
  line L3567 (19.2993, 26.6366) -> (19.2993, 25.6366)
  line L3568 (19.6422, 25.6366) -> (20.6422, 25.6366)
  line L3569 (20.6422, 25.6366) -> (20.6422, 26.6366)
  line L3570 (20.6422, 26.6366) -> (19.6422, 26.6366)
  line L3571 (19.6422, 26.6366) -> (19.6422, 25.6366)
  line L3572 (20.3407, 25.6366) -> (21.3407, 25.6366)
  line L3573 (21.3407, 25.6366) -> (21.3407, 26.6366)
  line L3574 (21.3407, 26.6366) -> (20.3407, 26.6366)
  line L3575 (20.3407, 26.6366) -> (20.3407, 25.6366)
  line L3576 (21.1281, 25.6366) -> (22.1281, 25.6366)
  line L3577 (22.1281, 25.6366) -> (22.1281, 26.6366)
  line L3578 (22.1281, 26.6366) -> (21.1281, 26.6366)
  line L3579 (21.1281, 26.6366) -> (21.1281, 25.6366)
  line L3580 (21.9409, 25.6366) -> (22.9409, 25.6366)
  line L3581 (22.9409, 25.6366) -> (22.9409, 26.6366)
  line L3582 (22.9409, 26.6366) -> (21.9409, 26.6366)
  line L3583 (21.9409, 26.6366) -> (21.9409, 25.6366)
  line L3584 (12.6191, 25.662) -> (13.6191, 25.662)
  line L3585 (13.6191, 25.662) -> (13.6191, 26.662)
  line L3586 (13.6191, 26.662) -> (12.6191, 26.662)
  line L3587 (12.6191, 26.662) -> (12.6191, 25.662)
  line L3588 (13.2033, 25.662) -> (14.2033, 25.662)
  line L3589 (14.2033, 25.662) -> (14.2033, 26.662)
  line L3590 (14.2033, 26.662) -> (13.2033, 26.662)
  line L3591 (13.2033, 26.662) -> (13.2033, 25.662)
  line L3592 (14.3336, 25.662) -> (15.3336, 25.662)
  line L3593 (15.3336, 25.662) -> (15.3336, 26.662)
  line L3594 (15.3336, 26.662) -> (14.3336, 26.662)
  line L3595 (14.3336, 26.662) -> (14.3336, 25.662)
  line L3596 (14.9305, 25.662) -> (15.9305, 25.662)
  line L3597 (15.9305, 25.662) -> (15.9305, 26.662)
  line L3598 (15.9305, 26.662) -> (14.9305, 26.662)
  line L3599 (14.9305, 26.662) -> (14.9305, 25.662)
  line L3600 (15.7941, 25.662) -> (16.7941, 25.662)
  line L3601 (16.7941, 25.662) -> (16.7941, 26.662)
  line L3602 (16.7941, 26.662) -> (15.7941, 26.662)
  line L3603 (15.7941, 26.662) -> (15.7941, 25.662)
  line L3604 (17.1149, 25.662) -> (18.1149, 25.662)
  line L3605 (18.1149, 25.662) -> (18.1149, 26.662)
  line L3606 (18.1149, 26.662) -> (17.1149, 26.662)
  line L3607 (17.1149, 26.662) -> (17.1149, 25.662)
  line L3608 (17.9658, 25.662) -> (18.9658, 25.662)
  line L3609 (18.9658, 25.662) -> (18.9658, 26.662)
  line L3610 (18.9658, 26.662) -> (17.9658, 26.662)
  line L3611 (17.9658, 26.662) -> (17.9658, 25.662)
  line L3612 (18.5119, 25.662) -> (19.5119, 25.662)
  line L3613 (19.5119, 25.662) -> (19.5119, 26.662)
  line L3614 (19.5119, 26.662) -> (18.5119, 26.662)
  line L3615 (18.5119, 26.662) -> (18.5119, 25.662)
  line L3616 (19.4644, 25.662) -> (20.4644, 25.662)
  line L3617 (20.4644, 25.662) -> (20.4644, 26.662)
  line L3618 (20.4644, 26.662) -> (19.4644, 26.662)
  line L3619 (19.4644, 26.662) -> (19.4644, 25.662)
  line L3620 (20.3407, 25.662) -> (21.3407, 25.662)
  line L3621 (21.3407, 25.662) -> (21.3407, 26.662)
  line L3622 (21.3407, 26.662) -> (20.3407, 26.662)
  line L3623 (20.3407, 26.662) -> (20.3407, 25.662)
  line L3624 (21.1281, 25.662) -> (22.1281, 25.662)
  line L3625 (22.1281, 25.662) -> (22.1281, 26.662)
  line L3626 (22.1281, 26.662) -> (21.1281, 26.662)
  line L3627 (21.1281, 26.662) -> (21.1281, 25.662)
  line L3628 (21.9536, 25.662) -> (22.9536, 25.662)
  line L3629 (22.9536, 25.662) -> (22.9536, 26.662)
  line L3630 (22.9536, 26.662) -> (21.9536, 26.662)
  line L3631 (21.9536, 26.662) -> (21.9536, 25.662)
  line L3632 (12.6445, 25.6874) -> (13.6445, 25.6874)
  line L3633 (13.6445, 25.6874) -> (13.6445, 26.6874)
  line L3634 (13.6445, 26.6874) -> (12.6445, 26.6874)
  line L3635 (12.6445, 26.6874) -> (12.6445, 25.6874)
  line L3636 (13.2287, 25.6874) -> (14.2287, 25.6874)
  line L3637 (14.2287, 25.6874) -> (14.2287, 26.6874)
  line L3638 (14.2287, 26.6874) -> (13.2287, 26.6874)
  line L3639 (13.2287, 26.6874) -> (13.2287, 25.6874)
  line L3640 (14.359, 25.6874) -> (15.359, 25.6874)
  line L3641 (15.359, 25.6874) -> (15.359, 26.6874)
  line L3642 (15.359, 26.6874) -> (14.359, 26.6874)
  line L3643 (14.359, 26.6874) -> (14.359, 25.6874)
  line L3644 (14.9559, 25.6874) -> (15.9559, 25.6874)
  line L3645 (15.9559, 25.6874) -> (15.9559, 26.6874)
  line L3646 (15.9559, 26.6874) -> (14.9559, 26.6874)
  line L3647 (14.9559, 26.6874) -> (14.9559, 25.6874)
  line L3648 (15.7814, 25.6874) -> (16.7814, 25.6874)
  line L3649 (16.7814, 25.6874) -> (16.7814, 26.6874)
  line L3650 (16.7814, 26.6874) -> (15.7814, 26.6874)
  line L3651 (15.7814, 26.6874) -> (15.7814, 25.6874)
  line L3652 (17.1022, 25.6874) -> (18.1022, 25.6874)
  line L3653 (18.1022, 25.6874) -> (18.1022, 26.6874)
  line L3654 (18.1022, 26.6874) -> (17.1022, 26.6874)
  line L3655 (17.1022, 26.6874) -> (17.1022, 25.6874)
  line L3656 (17.9658, 25.6874) -> (18.9658, 25.6874)
  line L3657 (18.9658, 25.6874) -> (18.9658, 26.6874)
  line L3658 (18.9658, 26.6874) -> (17.9658, 26.6874)
  line L3659 (17.9658, 26.6874) -> (17.9658, 25.6874)
  line L3660 (18.5119, 25.6874) -> (19.5119, 25.6874)
  line L3661 (19.5119, 25.6874) -> (19.5119, 26.6874)
  line L3662 (19.5119, 26.6874) -> (18.5119, 26.6874)
  line L3663 (18.5119, 26.6874) -> (18.5119, 25.6874)
  line L3664 (19.4644, 25.6874) -> (20.4644, 25.6874)
  line L3665 (20.4644, 25.6874) -> (20.4644, 26.6874)
  line L3666 (20.4644, 26.6874) -> (19.4644, 26.6874)
  line L3667 (19.4644, 26.6874) -> (19.4644, 25.6874)
  line L3668 (20.3407, 25.6874) -> (21.3407, 25.6874)
  line L3669 (21.3407, 25.6874) -> (21.3407, 26.6874)
  line L3670 (21.3407, 26.6874) -> (20.3407, 26.6874)
  line L3671 (20.3407, 26.6874) -> (20.3407, 25.6874)
  line L3672 (21.1154, 25.6874) -> (22.1154, 25.6874)
  line L3673 (22.1154, 25.6874) -> (22.1154, 26.6874)
  line L3674 (22.1154, 26.6874) -> (21.1154, 26.6874)
  line L3675 (21.1154, 26.6874) -> (21.1154, 25.6874)
  line L3676 (21.9663, 25.6874) -> (22.9663, 25.6874)
  line L3677 (22.9663, 25.6874) -> (22.9663, 26.6874)
  line L3678 (22.9663, 26.6874) -> (21.9663, 26.6874)
  line L3679 (21.9663, 26.6874) -> (21.9663, 25.6874)
  line L3680 (12.6699, 25.7128) -> (13.6699, 25.7128)
  line L3681 (13.6699, 25.7128) -> (13.6699, 26.7128)
  line L3682 (13.6699, 26.7128) -> (12.6699, 26.7128)
  line L3683 (12.6699, 26.7128) -> (12.6699, 25.7128)
  line L3684 (14.3844, 25.7128) -> (15.3844, 25.7128)
  line L3685 (15.3844, 25.7128) -> (15.3844, 26.7128)
  line L3686 (15.3844, 26.7128) -> (14.3844, 26.7128)
  line L3687 (14.3844, 26.7128) -> (14.3844, 25.7128)
  line L3688 (14.9813, 25.7128) -> (15.9813, 25.7128)
  line L3689 (15.9813, 25.7128) -> (15.9813, 26.7128)
  line L3690 (15.9813, 26.7128) -> (14.9813, 26.7128)
  line L3691 (14.9813, 26.7128) -> (14.9813, 25.7128)
  line L3692 (15.756, 25.7128) -> (16.756, 25.7128)
  line L3693 (16.756, 25.7128) -> (16.756, 26.7128)
  line L3694 (16.756, 26.7128) -> (15.756, 26.7128)
  line L3695 (15.756, 26.7128) -> (15.756, 25.7128)
  line L3696 (17.1022, 25.7128) -> (18.1022, 25.7128)
  line L3697 (18.1022, 25.7128) -> (18.1022, 26.7128)
  line L3698 (18.1022, 26.7128) -> (17.1022, 26.7128)
  line L3699 (17.1022, 26.7128) -> (17.1022, 25.7128)
  line L3700 (17.9658, 25.7128) -> (18.9658, 25.7128)
  line L3701 (18.9658, 25.7128) -> (18.9658, 26.7128)